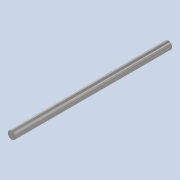
# Autodesk Inventor part: 0005-10-1018 tija 8
Saved by Autodesk Inventor 2020 (Build 240168000, 168)
## iProperties
Created: 2020-12-20
Part Number: 0005-10-1018 tija 8
Material: Stainless Steel
Document SubType Name: Modeling
Designer: Iulian Bors
Density: 8 g/cm^3
Appearance: Semi-Polished
Mass: 65.5462 g
Surface Area: 41.9717 cm^2
Volume: 8.19327 cm^3
Author: Iulian Bors
Subject: 10-1018
Autodesk Inventor part; units mm, degrees
ref_plane "YZ Plane" through (0, 0, 0) normal (1, 0, 0) x (0, 1, 0)
ref_plane "XZ Plane" through (0, 0, 0) normal (0, 1, 0) x (-1, 0, 0)
ref_plane "XY Plane" through (0, 0, 0) normal (0, 0, 1) x (1, 0, 0)
sketch "Sketch1" plane through (0, 0, 0) normal (0, 0, 1) x (1, 0, 0)
  circle A0 centre (0, 0) radius 4
  dimension "d0" = 8
  constraints: 1 centre point, 1 coincident
  measures "d0" diameter of A0
extrude "Extrusion1" add sketch "Sketch1" along normal blind 163
body "Solid1"
